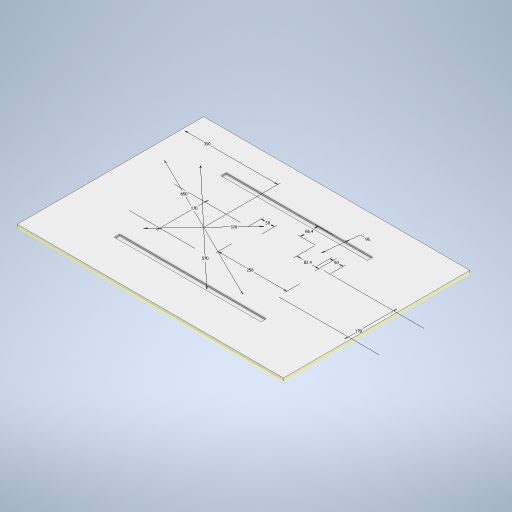
# Autodesk Inventor part: Base Plate Demo
Saved by Autodesk Inventor 2023 (Build 270158000, 158)
## iProperties
Created: 2023-02-23
Part Number: Base Plate Demo
Material: Acetal Resin, White
Document SubType Name: Modeling
Designer: cheng
Density: 1.425 g/cm^3
Appearance: Smooth - White
Author: cheng
Autodesk Inventor part; units mm, degrees
ref_plane "YZ Plane" through (0, 0, 0) normal (1, 0, 0) x (0, 1, 0)
ref_plane "XZ Plane" through (0, 0, 0) normal (0, 1, 0) x (-1, 0, 0)
ref_plane "XY Plane" through (0, 0, 0) normal (0, 0, 1) x (1, 0, 0)
sketch "Sketch1" plane through (0, 0, 0) normal (0, 1, 0) x (-1, 0, 0)
  line L0 (500, -350) -> (-500, -350)
  line L1 (-500, -350) -> (-500, 350)
  line L2 (-500, 350) -> (500, 350)
  line L3 (500, 350) -> (500, -350)
  line L4 (500, -350) -> (-500, 350) construction
  line L5 (-500, -350) -> (500, 350) construction
  point P0 (0, 0)
  dimension "d0" = 1000
  dimension "d1" = 700
  constraints: 12 end point, 2 midpoint, 2 parallel, 1 horizontal, 1 perpendicular
  measures "d0" distance between parallel lines of L1 L3
  measures "d1" distance between parallel lines of L2 L0
extrude "Extrusion1" add sketch "Sketch1" along normal blind 10
sketch "Sketch2" plane through (0, 10, 0) normal (0, 1, 0) x (1, 0, 0)
  line L0 (-500, -350) -> (500, -350) projected
  line L1 (500, -350) -> (500, 350) projected
  line L2 (500, 350) -> (-500, 350) projected
  line L3 (-500, 350) -> (-500, -350) projected
  line L4 (-275, -210) -> (275, -210) construction
  line L5 (275, -210) -> (275, 210) construction
  line L6 (275, 210) -> (-275, 210) construction
  line L7 (-275, 210) -> (-275, -210) construction
  line L8 (-275, -210) -> (275, 210) construction
  line L9 (275, -210) -> (-275, 210) construction
  line L10 (-275, -210) -> (275, -210)
  line L11 (275, -210) -> (275, -190)
  line L12 (275, -190) -> (-275, -190)
  line L13 (-275, -190) -> (-275, -210)
  line L14 (-275, 210) -> (275, 210)
  line L15 (275, 210) -> (275, 190)
  line L16 (275, 190) -> (-275, 190)
  line L17 (-275, 190) -> (-275, 210)
  point P0 (0, 0)
  dimension "d4" = 550
  dimension "d5" = 420
  dimension "d6" = 20
  dimension "d7" = 20
  constraints: 28 end point, 6 parallel, 3 horizontal, 3 perpendicular, 2 midpoint, 2 point on line
  measures "d4" distance of L6.end L5.end
  measures "d5" distance of L5.end L4.end
  measures "d6" distance of L11.end L10.end
  measures "d7" distance of L14.end L15.end
extrude "Extrusion2" cut sketch "Sketch2" against normal blind 5 contours L13 L12 L11 L10 | L14 L15 L16 L17
sketch "Sketch3" plane through (0, 0, 0) normal (0, -1, 0) x (1, 0, 0)
  line L0 (-500, 350) -> (500, 350) projected
  line L1 (-500, -350) -> (-500, 350) projected
  line L2 (500, -350) -> (-500, -350) projected
  line L3 (500, 350) -> (500, -350) projected
  line L4 (500, -350) -> (-500, -350) construction
  line L5 (0, -350) -> (0, 350) construction
  line L6 (-500, -350) -> (-500, 350) construction
  line L7 (-500, 0) -> (500, 0) construction
  circle A0 centre (-150, 0) radius 285
  circle A1 centre (-150, 0) radius 325 construction
  line L8 (200.7977, -218.4266) -> (118.3977, -218.4266)
  line L9 (118.3977, -218.4266) -> (118.3977, -152.0266)
  line L10 (118.3977, -152.0266) -> (200.7977, -152.0266)
  line L11 (200.7977, -152.0266) -> (200.7977, -218.4266)
  line L12 (-18.9239, 85) -> (-68.9239, 85)
  line L13 (-68.9239, 85) -> (-68.9239, -85)
  line L14 (-68.9239, -85) -> (-18.9239, -85)
  line L15 (-18.9239, -85) -> (-18.9239, 85)
  line L16 (239.0761, 85) -> (189.0761, 85)
  line L17 (189.0761, 85) -> (189.0761, -85)
  line L18 (189.0761, -85) -> (239.0761, -85)
  line L19 (239.0761, -85) -> (239.0761, 85)
  circle A2 centre (-150, 0) radius 160 construction
  line L20 (200.7977, -152.0266) -> (118.3977, -218.4266) construction
  line L21 (118.3977, -152.0266) -> (200.7977, -218.4266) construction
  circle A3 centre (159.5977, -185.2266) radius 48 construction
  line L22 (239.0761, -85) -> (189.0761, 85) construction
  line L23 (239.0761, 85) -> (189.0761, -85) construction
  line L24 (-18.9239, -85) -> (-68.9239, 85) construction
  line L25 (-18.9239, 85) -> (-68.9239, -85) construction
  line L26 (214.0761, 0) -> (-43.9239, 0) construction
  point P0 (0, 0)
  point P1 (85.0761, 0)
  dimension "d10" = 570
  dimension "d11" = 650
  dimension "d12" = 82.4
  dimension "d13" = 66.4
  dimension "d14" = 50
  dimension "d15" = 170
  dimension "d16" = 50
  dimension "d17" = 170
  dimension "d18" = 320
  dimension "d19" = 350
  dimension "d20" = 96
  dimension "d21" = 258
  constraints: 42 end point, 8 midpoint, 6 parallel, 4 centre point, 4 horizontal, 3 coincident, 3 perpendicular, 2 point on line, 2 other
  measures "d10" diameter of A0
  measures "d11" diameter of A1
  measures "d12" distance of L9.end L10.end
  measures "d13" distance of L8.end L9.end
  measures "d14" distance of L14.end L13.end
  measures "d15" distance of L13.end L12.end
  measures "d16" distance of L18.end L17.end
  measures "d17" distance of L17.end L17.start
  measures "d18" diameter of A2
  measures "d19" distance from line of L1 A0.centre
  measures "d20" diameter of A3
  measures "d21" distance of L26.start L26.end
extrude "Extrusion3" cut sketch "Sketch3" against normal blind 1 contours A0 | L8 L9 L10 L11
extrude "Extrusion4" cut sketch "Sketch3" against normal blind 2 contours L15 L14 L13 L12 | L19 L18 L17 L16
extrude "Extrusion5" cut sketch "Sketch3" against normal blind 0.1 contours A0 | L8 L9 L10 L11
extrude "Extrusion6" cut sketch "Sketch3" against normal blind 1 contours A0 | L8 L9 L10 L11
extrude "Extrusion7" cut sketch "Sketch3" against normal blind 2 contours A0 | L8 L9 L10 L11
extrude "Extrusion8" cut sketch "Sketch3" against normal blind 3 contours L15 L14 L13 L12 | L19 L18 L17 L16
body "Solid1"
